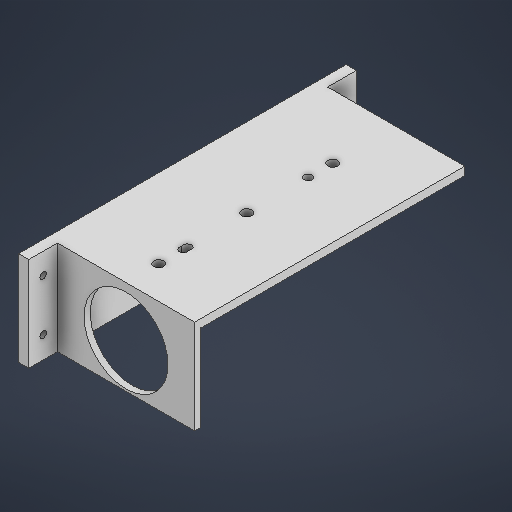
# Autodesk Inventor part: Laser Bracket
Saved by Autodesk Inventor 2025 (Build 290162000, 162)
## iProperties
Created: 2024-04-26
Part Number: Laser Bracket
Material: Generic
Document SubType Name: Modeling
Designer: Thienan Hoang
Density: 1 g/cm^3
Appearance: Default
Author: Thienan Hoang
Autodesk Inventor part; units mm, degrees
ref_plane "YZ Plane" through (0, 0, 0) normal (1, 0, 0) x (0, 1, 0)
ref_plane "XZ Plane" through (0, 0, 0) normal (0, 1, 0) x (-1, 0, 0)
ref_plane "XY Plane" through (0, 0, 0) normal (0, 0, 1) x (1, 0, 0)
sketch "Sketch1" plane through (0, 0, 0) normal (0, 1, 0) x (-1, 0, 0)
  line L0 (33.5, 64.5) -> (-33.5, 64.5)
  line L1 (-33.5, 64.5) -> (-33.5, -64.5)
  line L2 (-33.5, -64.5) -> (33.5, -64.5)
  line L3 (33.5, -64.5) -> (33.5, 64.5)
  line L4 (33.5, 64.5) -> (-33.5, -64.5) construction
  line L5 (-33.5, 64.5) -> (33.5, -64.5) construction
  point P0 (0, 0)
  dimension "d0" = 67
  dimension "d1" = 129
  constraints: 12 end point, 2 midpoint, 2 parallel, 1 horizontal, 1 perpendicular
  measures "d0" distance of L2.end L1.end
  measures "d1" distance of L1.end L0.end
extrude "Extrusion1" add sketch "Sketch1" along normal blind 3
sketch "Sketch2" plane through (0, 0, 0) normal (0, -1, 0) x (1, 0, 0)
  circle A0 centre (0, 51.5) radius 3
  line L0 (-2, 39.5) -> (-2, 37.5)
  line L1 (2, 37.5) -> (2, 39.5)
  circle A1 centre (0, 8.5) radius 3.487
  circle A2 centre (0, -21.5) radius 2
  circle A3 centre (0, -33.5) radius 3
  arc A4 (2, 39.5) -> (-2, 39.5) centre (0, 39.5) ccw
  arc A5 (-2, 37.5) -> (2, 37.5) centre (0, 37.5) ccw
  line L2 (-33.5, 64.5) -> (33.5, 64.5) projected
  point P0 (0, 0)
  point P1 (2, 38.5)
  point P2 (-2, 38.5)
  dimension "d4" = 6
  dimension "d7" = 4
  dimension "d8" = 6
  dimension "d9" = 13
  dimension "d10" = 56
  dimension "d11" = 26
  dimension "d12" = 60
  dimension "d13" = 85
  constraints: 6 centre point, 4 end point, 4 point on circle, 2 midpoint, 1 parallel
  measures "d4" diameter of A0
  measures "d7" diameter of A2
  measures "d8" diameter of A3
  measures "d9" distance from line of L2 A0.centre
  measures "d10" distance from line of L2 A1.centre
  measures "d11" distance from line of L2 point (2, 38.5)
  measures "d12" vertical distance of A2.centre point (-2, 38.5)
  measures "d13" distance of A3.centre A0.centre
hole "Hole1" at (0, 0, 51.5) at (0, 0, -33.5) direction (0, 1, 0) diameter 4.917 depth 17.1 thread size "M6x1" class "6H" standard "ANSI Metric M Profile"
hole "Hole2" at (0, 0, -21.5) at (0, 0, 39.5) at (0, 0, 37.5) direction (0, 1, 0) diameter 4 depth 17.1
hole "Hole3" at (0, 0, 8.5) direction (0, 1, 0) diameter 4.9784 depth 19.05 thread size "1/4-20 UNC" class "2B" standard "ANSI Unified Screw Threads"
sketch "Sketch3" plane through (-33.5, 0, 64.5) normal (0, 0, 1) x (1, 0, 0)
  line L0 (0, 3) -> (67, 3) projected
  line L1 (0, 3) -> (67, 3)
  line L2 (67, 3) -> (67, 0)
  line L3 (67, 0) -> (0, 0)
  line L4 (0, 0) -> (0, 3)
  point P0 (33.5, 0)
  constraints: 8 end point, 2 parallel, 1 horizontal, 1 perpendicular
extrude "Extrusion2" add sketch "Sketch3" along normal blind 3
sketch "Sketch4" plane through (0, 3, 0) normal (0, 1, 0) x (1, 0, 0)
  line L0 (-33.5, 64.5) -> (-33.5, -67.5) projected
  line L1 (33.5, 64.5) -> (33.5, -67.5) projected
  line L2 (-33.5, -67.5) -> (33.5, -67.5)
  line L3 (33.5, -67.5) -> (33.5, -64.5)
  line L4 (33.5, -64.5) -> (-33.5, -64.5)
  line L5 (-33.5, -64.5) -> (-33.5, -67.5)
  point P0 (0, 0)
  point P1 (-33.5, -64.5)
  dimension "d37" = 3
  constraints: 8 end point, 2 parallel, 1 horizontal, 1 perpendicular, 1 point on line
  measures "d37" distance of L3.end L2.end
extrude "Extrusion3" add sketch "Sketch4" along normal blind 45
sketch "Sketch5" plane through (-33.5, 0, 67.5) normal (0, 0, 1) x (1, 0, 0)
  circle A0 centre (33.5, 23.5) radius 20.5
  line L0 (0, 0) -> (67, 0) projected
  line L1 (0, 48) -> (67, 48) projected
  point P0 (33.5, 0)
  point P1 (33.5, 48)
  dimension "d40" = 41
  dimension "d41" = 23.5
  constraints: 1 centre point, 1 midpoint, 1 vertical alignment
  measures "d40" diameter of A0
  measures "d41" distance from line of L0 A0.centre
extrude "Extrusion4" cut sketch "Sketch5" against normal blind 45
sketch "Sketch6" plane through (-33.5, 0, -64.5) normal (-1, 0, 0) x (0, 0, 1)
  line L0 (0, 0) -> (0, 3) projected
  line L1 (132, 0) -> (0, 0) projected
  line L2 (0, 3) -> (132, 3)
  line L3 (132, 3) -> (132, 0)
  line L4 (132, 0) -> (0, 0)
  line L5 (0, 0) -> (0, 3)
  point P0 (64.5, 0)
  constraints: 8 end point, 2 parallel, 1 horizontal, 1 perpendicular
extrude "Extrusion5" add sketch "Sketch6" along normal blind 5
sketch "Sketch7" plane through (0, 3, 0) normal (0, 1, 0) x (1, 0, 0)
  line L0 (33.5, -67.5) -> (-38.5, -67.5) projected
  line L1 (33.5, 64.5) -> (-38.5, 64.5) projected
  line L2 (-38.5, -67.5) -> (-33.5, -67.5)
  line L3 (-33.5, -67.5) -> (-33.5, 64.5)
  line L4 (-33.5, 64.5) -> (-38.5, 64.5)
  line L5 (-38.5, 64.5) -> (-38.5, -67.5)
  point P0 (0, 0)
  point P1 (-38.5, 64.5)
  dimension "d46" = 5
  constraints: 8 end point, 2 parallel, 1 horizontal, 1 perpendicular, 1 point on line
  measures "d46" distance of L4.end L3.end
extrude "Extrusion6" add sketch "Sketch7" along normal blind 45
sketch "Sketch8" plane through (33.5, 0, -64.5) normal (0, 0, -1) x (-1, 0, 0)
  line L0 (0, 48) -> (67, 48) projected
  line L1 (72, 0) -> (72, 48) projected
  line L2 (67, 48) -> (72, 48)
  line L3 (72, 48) -> (72, 0)
  line L4 (72, 0) -> (67, 0)
  line L5 (67, 0) -> (67, 48)
  point P0 (33.5, 0)
  constraints: 8 end point, 2 parallel, 1 horizontal, 1 perpendicular
extrude "Extrusion7" add sketch "Sketch8" along normal blind 14
sketch "Sketch9" plane through (-33.5, 0, 67.5) normal (0, 0, 1) x (1, 0, 0)
  line L0 (-5, 0) -> (-5, 48) projected
  line L1 (67, 0) -> (-5, 0) projected
  line L2 (-5, 48) -> (0, 48)
  line L3 (0, 48) -> (0, 0)
  line L4 (0, 0) -> (-5, 0)
  line L5 (-5, 0) -> (-5, 48)
  point P0 (33.5, 0)
  dimension "d51" = 5
  constraints: 8 end point, 2 parallel, 1 horizontal, 1 perpendicular, 1 point on line
  measures "d51" distance of L3.end L4.end
extrude "Extrusion8" add sketch "Sketch9" along normal blind 14
sketch "Sketch10" plane through (0, 0, 0) normal (0, -1, 0) x (1, 0, 0)
  line L0 (-33.5, 64.5) -> (-33.5, -78.5) projected
  line L1 (-38.5, 81.5) -> (-33.5, 81.5) projected
  line L2 (-33.5, -78.5) -> (-38.5, -78.5)
  line L3 (-38.5, -78.5) -> (-38.5, 81.5)
  line L4 (-38.5, 81.5) -> (-33.5, 81.5)
  line L5 (-33.5, 81.5) -> (-33.5, -78.5)
  point P0 (0, 0)
  constraints: 8 end point, 2 parallel, 1 horizontal, 1 perpendicular
sketch "Sketch11" plane through (-33.5, 3, 64.5) normal (1, 0, 0) x (0, 0, -1)
  circle A0 centre (136, 9.75) radius 2
  circle A1 centre (135.5136, 34.75) radius 2
  line L0 (143, -5) -> (-17, -5) projected
  line L1 (143, 45) -> (143, -3) projected
  circle A2 centre (-10, 9.75) radius 2
  circle A3 centre (-10, 34.75) radius 2
  line L2 (-17, 45) -> (-17, -5) projected
  point P0 (64.5, -3)
  dimension "d56" = 4
  dimension "d57" = 4
  dimension "d58" = 14.75
  dimension "d59" = 7
  dimension "d60" = 25
  dimension "d68" = 4
  dimension "d69" = 14.75
  dimension "d70" = 7
  dimension "d71" = 7
  dimension "d72" = 25
  constraints: 4 centre point
  measures "d56" diameter of A0
  measures "d57" diameter of A1
  measures "d58" distance from line of L0 A0.centre
  measures "d59" distance from line of L1 A0.centre
  measures "d60" vertical distance of A1.centre A0.centre
  measures "d68" diameter of A2
  measures "d69" distance from line of L0 A2.centre
  measures "d70" distance from line of L2 A2.centre
  measures "d71" distance from line of L2 A3.centre
  measures "d72" distance of A2.centre A3.centre
hole "Hole4" at (-33.5, 37.75, -71.0136) at (-33.5, 12.75, -71.5) at (-33.5, 37.75, 74.5) at (-33.5, 12.75, 74.5) direction (-1, 0, 0) diameter 3.242 depth 10 tip angle 118 thread size "M4x0.7" class "6H" standard "ANSI Metric M Profile"
sketch "Sketch12" plane through (-33.5, 3, 64.5) normal (1, 0, 0) x (0, 0, -1)
  line L0 (-3, 45) -> (0, 45) projected
  line L1 (0, 45) -> (129, 45)
  line L2 (129, 45) -> (129, 41)
  line L3 (129, 41) -> (0, 41)
  line L4 (0, 41) -> (0, 45)
  point P0 (64.5, -3)
  dimension "d73" = 129
  dimension "d74" = 4
  constraints: 8 end point, 2 parallel, 1 horizontal, 1 perpendicular
  measures "d73" distance of L2.end L3.end
  measures "d74" distance of L1.end L2.end
extrude "Extrusion10" add sketch "Sketch12" along normal up to surface (67 mm away)
hole "Hole5" at (0, 0, 51.5) at (0, 0, -33.5) direction (0, 1, 0) diameter 4.917 end through all thread size "M6x1" class "6H" standard "ANSI Metric M Profile"
hole "Hole6" at (0, 0, 8.5) direction (0, 1, 0) diameter 4.9784 end through all thread size "1/4-20 UNC" class "2B" standard "ANSI Unified Screw Threads"
hole "Hole7" at (0, 0, -21.5) at (0, 0, 39.5) at (0, 0, 37.5) direction (0, 1, 0) diameter 4 end through all
sketch "Sketch13" plane through (0, 3, 0) normal (0, 1, 0) x (1, 0, 0)
  line L0 (-33.5, 64.5) -> (-33.5, -64.5) projected
  line L1 (33.5, 64.5) -> (-33.5, 64.5) projected
  line L2 (-33.5, -64.5) -> (33.5, -64.5)
  line L3 (33.5, -64.5) -> (33.5, 64.5)
  line L4 (33.5, 64.5) -> (-33.5, 64.5)
  line L5 (-33.5, 64.5) -> (-33.5, -64.5)
  point P0 (0, 0)
  constraints: 8 end point, 2 parallel, 1 horizontal, 1 perpendicular
extrude "Extrusion11" cut sketch "Sketch13" against normal blind 10
sketch "Sketch14" plane through (0, 0, 0) normal (0, -1, 0) x (1, 0, 0)
  line L0 (58.5292, 135.8199) -> (-75.2061, 135.8199)
  line L1 (-75.2061, 135.8199) -> (-75.2061, -131.0093)
  line L2 (-75.2061, -131.0093) -> (58.5292, -131.0093)
  line L3 (58.5292, -131.0093) -> (58.5292, 135.8199)
  point P0 (0, 0)
  constraints: 8 end point, 2 parallel, 1 horizontal, 1 perpendicular
extrude "Extrusion12" cut sketch "Sketch14" against normal blind 2
body "Solid1"
